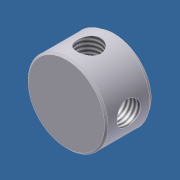
# Autodesk Inventor part: Regulator Base 1764
Saved by Autodesk Inventor 2011 (Build 150239000, 239)
## iProperties
Created: 2010-02-17
Part Number: Regulator Base 1764
Document SubType Name: Modeling
Designer: jgehrig
Density: 1 g/cm^3
Author: jgehrig
Autodesk Inventor part; units mm, degrees
sketch "Sketch1" plane through (0, 0, 0) normal (0, 0, 1) x (1, 0, 0)
  circle A0 centre (0, 0) radius 18.0975
  dimension "d0" = 36.195
  constraints: 1 centre point, 1 coincident
  measures "d0" diameter of A0
extrude "Extrusion1" add sketch "Sketch1" along normal blind 19.685
chamfer "Chamfer1" distance 0.7937 angle 45 1 edges at (-18.0975, 0, 19.685)
sketch "Sketch2" plane through (0, 0, 0) normal (0, 0, -1) x (-1, 0, 0)
  circle A0 centre (0, 0) radius 18.0975 projected
  circle A1 centre (0, 0) radius 16.8275
  dimension "d6" = 33.655
  constraints: 1 centre point, 1 coincident
  measures "d6" diameter of A1
extrude "Extrusion2" add sketch "Sketch2" along normal blind 1.905 contours A1
ref_plane "Work Plane1" through (0, 0, 0) normal (0, 1, 0) x (-1, 0, 0)
sketch "Sketch3" plane through (0, 0, 0) normal (0, 1, 0) x (-1, 0, 0)
  line L0 (-18.0975, 0) -> (18.0975, 0) projected
  line L1 (18.0975, 18.8913) -> (-18.0975, 18.8913) projected
  line L2 (18.0975, 0) -> (18.0975, 18.8913) projected
  line L3 (-18.0975, 0) -> (-18.0975, 18.8913) projected
  circle A0 centre (0, 9.4456) radius 5.3975
  point P0 (0, 0)
  dimension "d10" = 10.795
  constraints: 1 centre point
  measures "d10" diameter of A0
extrude "Extrusion3" cut sketch "Sketch3" against normal mid plane 76.2 contours A0
ref_plane "Work Plane2" through (0, 0, 0) normal (0, 1, 0) x (-1, 0, 0)
sketch "Sketch4" plane through (0, 0, 0) normal (0, 1, 0) x (-1, 0, 0)
  point P0 (0, 0)
ref_plane "Work Plane3" through (0, 0, 0) normal (1, 0, 0) x (0, 1, 0)
sketch "Sketch5" plane through (0, 0, 0) normal (1, 0, 0) x (0, 1, 0)
  line L0 (18.0975, 0) -> (18.0975, 18.8913) projected
  line L1 (-18.0975, 0) -> (-18.0975, 18.8913) projected
  line L2 (-18.0975, 0) -> (18.0975, 0) projected
  line L3 (-17.3038, 19.685) -> (17.3038, 19.685) projected
  circle A0 centre (0, 9.4456) radius 5.3975
  point P0 (0, 0)
  dimension "d15" = 10.795
  constraints: 1 centre point
  measures "d15" diameter of A0
extrude "Extrusion4" cut sketch "Sketch5" against normal mid plane 76.2
thread "Thread1" size "7/16-14 UNC" class "2B" standard "ANSI Unified Screw Threads" full length
thread "Thread2" size "7/16-14 UNC" class "2B" standard "ANSI Unified Screw Threads" full length
thread "Thread3" size "7/16-14 UNC" class "2B" standard "ANSI Unified Screw Threads" full length
thread "Thread4" size "7/16-14 UNC" class "2B" standard "ANSI Unified Screw Threads" full length
body "Solid1"
